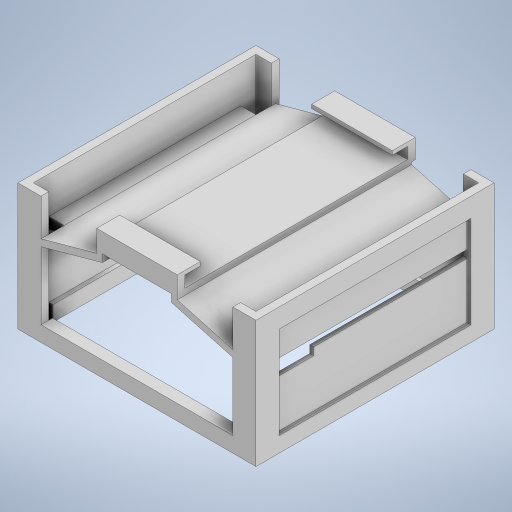
# Autodesk Inventor part: Unterbau V3
Saved by Autodesk Inventor 2023.1 (Build 271208000, 208)
## iProperties
Created: 2023-04-17
Part Number: Unterbau V3
Material: Generisch
Document SubType Name: Modeling
Designer: marco
Density: 1 g/cm^3
Appearance: Vorgabe
Author: marco
Autodesk Inventor part; units mm, degrees
ref_plane "YZ Plane" through (0, 0, 0) normal (1, 0, 0) x (0, 1, 0)
ref_plane "XZ Plane" through (0, 0, 0) normal (0, 1, 0) x (-1, 0, 0)
ref_plane "XY Plane" through (0, 0, 0) normal (0, 0, 1) x (1, 0, 0)
sketch "Skizze1" plane through (0, 0, 0) normal (0, 1, 0) x (-1, 0, 0)
  line L0 (0, 0) -> (62, 0)
  line L1 (62, 0) -> (62, -62)
  line L2 (62, -62) -> (0, -62)
  line L3 (0, -62) -> (0, 0)
  line L4 (2, -2) -> (6, -2)
  line L5 (6, -2) -> (6, -6)
  line L6 (6, -6) -> (2, -6)
  line L7 (2, -6) -> (2, -2)
  line L8 (2, -56) -> (6, -56)
  line L9 (6, -56) -> (6, -60)
  line L10 (6, -60) -> (2, -60)
  line L11 (2, -60) -> (2, -56)
  line L12 (56, -2) -> (60, -2)
  line L13 (60, -2) -> (60, -6)
  line L14 (60, -6) -> (56, -6)
  line L15 (56, -6) -> (56, -2)
  line L16 (56, -56) -> (60, -56)
  line L17 (60, -56) -> (60, -60)
  line L18 (60, -60) -> (56, -60)
  line L19 (56, -60) -> (56, -56)
  line L20 (3, -3) -> (59, -3)
  line L21 (59, -3) -> (59, -59)
  line L22 (59, -59) -> (3, -59)
  line L23 (3, -59) -> (3, -3)
  point P0 (2, -58)
  point P1 (6, -3)
  point P2 (56, -3)
  point P3 (59, -6)
  point P4 (59, -56)
  point P5 (56, -59)
  point P6 (6, -59)
  point P7 (3, -56)
  point P8 (3, -6)
  dimension "d0" = 62
  dimension "d1" = 62
  dimension "d2" = 4
  dimension "d3" = 4
  dimension "d4" = 4
  dimension "d5" = 4
  dimension "d6" = 4
  dimension "d7" = 50
  dimension "d8" = 50
  dimension "d9" = 2
  dimension "d10" = 2
  dimension "d11" = 2
  dimension "d12" = 56
  dimension "d13" = 56
  constraints: 48 end point, 12 parallel, 7 point on line, 6 horizontal, 6 perpendicular, 1 midpoint
  measures "d0" distance of L1.end L2.end
  measures "d1" distance of L0.end L1.end
  measures "d2" distance of L5.end L6.end
  measures "d3" distance of L4.end L5.end
  measures "d4" distance of L9.end L10.end
  measures "d5" distance of L8.end L9.end
  measures "d6" distance of L13.end L14.end
  measures "d7" distance between parallel lines of L15 L5
  measures "d8" distance between parallel lines of L8 L6
  measures "d9" distance between parallel lines of L2 L10
  measures "d10" distance between parallel lines of L1 L17
  measures "d11" distance from line of L3 point (2, -58)
  measures "d12" distance of L21.end L22.end
  measures "d13" distance of L20.end L21.end
extrude "Extrusion1" add sketch "Skizze1" along normal blind 4
sketch "Skizze2" plane through (0, 4, 0) normal (0, 1, 0) x (1, 0, 0)
  line L0 (-2, 2) -> (-6, 2) projected
  line L1 (-3, 6) -> (-2, 6) projected
  line L2 (-6, 2) -> (-2, 2)
  line L3 (-2, 2) -> (-2, 6)
  line L4 (-2, 6) -> (-6, 6)
  line L5 (-6, 6) -> (-6, 2)
  line L6 (-62, 0) -> (0, 0) projected
  line L7 (0, 0) -> (0, 62) projected
  line L8 (-6, 0) -> (0, 0)
  line L9 (0, 0) -> (0, 6)
  line L10 (0, 6) -> (-6, 6)
  line L11 (-6, 6) -> (-6, 0)
  line L12 (0, 62) -> (-62, 62) projected
  line L13 (0, 55.9421) -> (-6, 55.9421)
  line L14 (-6, 55.9421) -> (-6, 62)
  line L15 (-6, 62) -> (0, 62)
  line L16 (0, 62) -> (0, 55.9421)
  line L17 (-6, 59) -> (-6, 60) projected
  line L18 (-6, 60) -> (-2, 60)
  line L19 (-2, 60) -> (-2, 56)
  line L20 (-2, 56) -> (-6, 56)
  line L21 (-6, 56) -> (-6, 60)
  line L22 (-62, 62) -> (-56, 62)
  line L23 (-56, 62) -> (-56, 55.9421)
  line L24 (-56, 55.9421) -> (-62, 55.9421)
  line L25 (-62, 55.9421) -> (-62, 62)
  line L26 (-60, 60) -> (-56, 60) projected
  line L27 (-60, 60) -> (-56, 60)
  line L28 (-56, 60) -> (-56, 55.9421)
  line L29 (-56, 55.9421) -> (-60, 55.9421)
  line L30 (-60, 55.9421) -> (-60, 60)
  line L31 (-62, 62) -> (-62, 0) projected
  line L32 (-62, 6) -> (-56, 6)
  line L33 (-56, 6) -> (-56, 0)
  line L34 (-56, 0) -> (-62, 0)
  line L35 (-62, 0) -> (-62, 6)
  line L36 (-56, 2) -> (-60, 2)
  line L37 (-60, 2) -> (-60, 6)
  line L38 (-60, 6) -> (-56, 6)
  line L39 (-56, 6) -> (-56, 2)
  constraints: 64 end point, 16 parallel, 16 point on line, 8 horizontal, 8 perpendicular
extrude "Extrusion2" add sketch "Skizze2" along normal blind 25 contours L3 L10 L7 L6 L11 L0 | L6 L31 L32 L37 L36 L33 | L13 L14 L20 L19 L18 L12 L7 | L25 L12 L23 L26 L30 L24
sketch "Skizze3" plane through (0, 29, 0) normal (0, 1, 0) x (1, 0, 0)
  line L0 (-62, 0) -> (0, 0) projected
  line L1 (0, 0) -> (-62, 0)
  line L2 (-62, 0) -> (-62, 62)
  line L3 (-62, 62) -> (0, 62)
  line L4 (0, 62) -> (0, 0)
  line L5 (-6, 6) -> (-56, 6)
  line L6 (-56, 6) -> (-56, 56)
  line L7 (-56, 56) -> (-6, 56)
  line L8 (-6, 56) -> (-6, 6)
  line L9 (-60, 2) -> (-60, 6) projected
  line L10 (-56, 6) -> (-60, 6)
  line L11 (-60, 6) -> (-60, 2)
  line L12 (-60, 2) -> (-56, 2)
  line L13 (-56, 2) -> (-56, 6)
  line L14 (-60, 60) -> (-56, 60) projected
  line L15 (-56, 56) -> (-60, 56)
  line L16 (-60, 56) -> (-60, 60)
  line L17 (-60, 60) -> (-56, 60)
  line L18 (-56, 60) -> (-56, 56)
  line L19 (-3, 56) -> (-6, 56) projected
  line L20 (-2, 60) -> (-2, 56) projected
  line L21 (-6, 56) -> (-2, 56)
  line L22 (-2, 56) -> (-2, 60)
  line L23 (-2, 60) -> (-6, 60)
  line L24 (-6, 60) -> (-6, 56)
  line L25 (-2, 2) -> (-6, 2) projected
  line L26 (-6, 6) -> (-2, 6)
  line L27 (-2, 6) -> (-2, 2)
  line L28 (-2, 2) -> (-6, 2)
  line L29 (-6, 2) -> (-6, 6)
  dimension "d18" = 50
  dimension "d19" = 50
  constraints: 48 end point, 12 parallel, 6 horizontal, 6 perpendicular
  measures "d18" distance of L6.end L7.end
  measures "d19" distance of L5.end L6.end
extrude "Extrusion3" add sketch "Skizze3" along normal blind 4
sketch "Skizze4" plane through (0, 29, 0) normal (0, -1, 0) x (1, 0, 0)
  line L0 (-6, -6) -> (-56, -6) projected
  line L1 (-6, -6) -> (-2, -6)
  line L2 (-2, -6) -> (-2, -56)
  line L3 (-2, -56) -> (-6, -56)
  line L4 (-6, -56) -> (-6, -6)
  line L5 (-6, -56) -> (-56, -56)
  line L6 (-56, -56) -> (-56, -60)
  line L7 (-56, -60) -> (-6, -60)
  line L8 (-6, -60) -> (-6, -56)
  line L9 (-56, -6) -> (-56, -2) projected
  line L10 (-56, -6) -> (-6, -6)
  line L11 (-6, -6) -> (-6, -2)
  line L12 (-6, -2) -> (-56, -2)
  line L13 (-56, -2) -> (-56, -6)
  line L14 (-60, -6) -> (-56, -6) projected
  line L15 (-56, -6) -> (-60, -6)
  line L16 (-60, -6) -> (-60, -56)
  line L17 (-60, -56) -> (-56, -56)
  line L18 (-56, -56) -> (-56, -6)
  point P0 (0, 0)
  dimension "d22" = 4
  dimension "d23" = 50
  dimension "d24" = 50
  dimension "d25" = 4
  dimension "d26" = 50
  dimension "d27" = 4
  dimension "d28" = 4
  dimension "d29" = 50
  constraints: 32 end point, 8 parallel, 4 horizontal, 4 perpendicular
  measures "d22" distance of L2.end L3.end
  measures "d23" distance of L1.end L2.end
  measures "d24" distance of L7.end L6.end
  measures "d25" distance of L6.end L5.end
  measures "d26" distance of L12.end L11.end
  measures "d27" distance of L11.end L10.end
  measures "d28" distance of L17.end L16.end
  measures "d29" distance of L16.end L15.end
extrude "Extrusion4" cut sketch "Skizze4" against normal blind 2 contours L1 L2 L3 L4 | L0 L9 L12 L11 | L18 L17 L16 L14 | L8 L7 L6 L5
sketch "Skizze5" plane through (0, 31, 0) normal (0, -1, 0) x (1, 0, 0)
  line L0 (-59, -59) -> (-3, -59)
  line L1 (-3, -59) -> (-3, -3)
  line L2 (-59, -3) -> (-59, -59)
  line L3 (-57.5, -4.5) -> (-57.5, -57.5)
  line L4 (-57.5, -57.5) -> (-4.5, -57.5)
  line L5 (-4.5, -57.5) -> (-4.5, -4.5)
  line L6 (-62, 0) -> (0, 0) projected
  line L7 (0, 0) -> (0, -62) projected
  line L8 (-60, -60) -> (-56, -60) projected
  line L9 (-2, -6) -> (-2, -2) projected
  line L10 (-60, -60) -> (-2, -60)
  line L11 (-2, -60) -> (-2, -2)
  line L12 (-2, -2) -> (-60, -2)
  line L13 (-60, -2) -> (-60, -60)
  dimension "d32" = 56
  dimension "d33" = 56
  dimension "d34" = 53
  dimension "d35" = 53
  dimension "d36" = 1.5
  dimension "d39" = 3
  constraints: 20 end point, 4 parallel, 2 horizontal, 2 perpendicular
  measures "d32" distance of L2.start L1.end
  measures "d33" distance of L1.end L0.end
  measures "d34" distance of L4.end L3.end
  measures "d35" distance of L3.end L3.start
  measures "d36" distance between parallel lines of L5 L1
  measures "d39" distance between parallel lines of L1 L7
extrude "Extrusion5" cut sketch "Skizze5" against normal blind 1
sketch "Skizze6" plane through (0, 32, 0) normal (0, -1, 0) x (1, 0, 0)
  line L0 (-60, -6) -> (-56, -6) projected
  line L1 (-56, -6) -> (-52, -6)
  line L2 (-6, -6) -> (-56, -6) projected
  line L3 (-52, -6) -> (-56, -10)
  line L4 (-56, -6) -> (-56, -56) projected
  line L5 (-56, -10) -> (-56, -6)
  line L6 (-6, -56) -> (-6, -6) projected
  line L7 (-6, -6) -> (-10, -6)
  line L8 (-6, -6) -> (-2, -6) construction
  line L9 (-10, -6) -> (-6, -10)
  line L10 (-6, -10) -> (-6, -6)
  line L11 (-6, -56) -> (-6, -60) projected
  line L12 (-6, -56) -> (-6, -52)
  line L13 (-6, -52) -> (-10, -56)
  line L14 (-56, -56) -> (-6, -56) projected
  line L15 (-56, -56) -> (-52, -56)
  line L16 (-56, -52) -> (-52, -56)
  line L17 (-56, -52) -> (-56, -56)
  point P0 (0, 0)
  dimension "d42" = 4
  dimension "d43" = 45
  dimension "d44" = 4
  dimension "d45" = 180
  constraints: 24 end point, 6 point on line, 4 collinear, 2 perpendicular, 1 horizontal
  measures "d42" distance of L0.end L1.end
  measures "d43" angle of L1 L3
  measures "d44" distance of L2.start L7.end
  measures "d45" angle of L7 L8
extrude "Extrusion6" add sketch "Skizze6" against normal blind 1 contours L1 L3 L4 | L2 L6 L9 | L16 L14 L4 | L6 L14 L13
sketch "Skizze7" plane through (-6, 4, -55.9421) normal (0, 0, 1) x (1, 0, 0)
  line L0 (3, 0) -> (0, 0) projected
  line L1 (0, 0) -> (4, 0)
  line L2 (4, 0) -> (4, 25)
  line L3 (4, 25) -> (0, 25)
  line L4 (0, 25) -> (0, 0)
  point P0 (6, -4)
  constraints: 8 end point, 2 parallel, 1 horizontal, 1 perpendicular
extrude "Extrusion7" cut sketch "Skizze7" against normal blind 1
sketch "Skizze10" plane through (0, 29, 0) normal (0, -1, 0) x (1, 0, 0)
  line L0 (-2, -6) -> (-2, -55.9421) projected
  line L1 (-6, -6) -> (-2, -6) projected
  line L2 (-2, -6) -> (-6, -6)
  line L3 (-6, -2) -> (-6, -6) projected
  line L4 (-6, -6) -> (-6, -2)
  line L5 (-56, -3) -> (-56, -2) projected
  line L6 (-6, -2) -> (-56, -2)
  line L7 (-56, -6) -> (-56, -2) projected
  line L8 (-56, -2) -> (-56, -6)
  line L9 (-60, -6) -> (-56, -6) projected
  line L10 (-56, -6) -> (-60, -6)
  line L11 (-60, -56) -> (-60, -60) projected
  line L12 (-60, -6) -> (-60, -56)
  line L13 (-56, -56) -> (-60, -56) projected
  line L14 (-60, -56) -> (-56, -56)
  line L15 (-56, -60) -> (-56, -56) projected
  line L16 (-56, -56) -> (-56, -60)
  line L17 (-6, -59) -> (-6, -60) projected
  line L18 (-56, -60) -> (-6, -60)
  line L19 (-6, -56) -> (-6, -60) projected
  line L20 (-6, -60) -> (-6, -56)
  line L21 (-3, -56) -> (-2, -56) projected
  line L22 (-6, -56) -> (-2, -56)
  line L23 (-2, -56) -> (-2, -6)
  line L24 (0, -6) -> (0, -55.9421) projected
  line L25 (-2, -6) -> (0, -6)
  line L26 (0, -6) -> (0, -56)
  line L27 (0, -56) -> (-2, -56)
  line L28 (-6, -62) -> (-56, -62) projected
  line L29 (-6, -60) -> (-6, -62)
  line L30 (-6, -62) -> (-56, -62)
  line L31 (-56, -62) -> (-56, -60)
  line L32 (-56, 0) -> (-6, 0) projected
  line L33 (-56, -2) -> (-56, 0)
  line L34 (-56, 0) -> (-6, 0)
  line L35 (-6, -2) -> (-6, 0) projected
  line L36 (-6, 0) -> (-6, -2)
  line L37 (-60, -6) -> (-62, -6)
  line L38 (-62, -62) -> (-62, 0) projected
  line L39 (-62, -56) -> (-62, -6)
  line L40 (-59, -6) -> (-59, -56) projected
  line L41 (-62, -56) -> (-60, -56)
  point P0 (0, 0)
  constraints: 48 end point, 11 perpendicular, 8 collinear, 2 horizontal, 2 point on line, 2 vertical, 1 parallel
extrude "Extrusion8" add sketch "Skizze10" along normal blind 1
sketch "Skizze11" plane through (0, 0, 0) normal (0, -1, 0) x (1, 0, 0)
  line L0 (-60, -60) -> (-56, -60) projected
  line L1 (-2, -6) -> (-2, -2) projected
  line L2 (-60, -60) -> (-2, -60)
  line L3 (-2, -60) -> (-2, -2)
  line L4 (-2, -2) -> (-60, -2)
  line L5 (-60, -2) -> (-60, -60)
  line L6 (-1, -1) -> (-61, -1)
  line L7 (-61, -1) -> (-61, -61)
  line L8 (-61, -61) -> (-1, -61)
  line L9 (-1, -61) -> (-1, -1)
  point P0 (0, 0)
  dimension "d52" = 60
  dimension "d53" = 60
  constraints: 16 end point, 4 parallel, 2 horizontal, 2 perpendicular
  measures "d52" distance of L8.end L7.end
  measures "d53" distance of L7.end L6.end
extrude "Extrusion9" add sketch "Skizze11" against normal blind 28
sketch "Skizze13" plane through (-56, 28, -1) normal (0, 0, 1) x (1, 0, 0)
  line L0 (0, -24) -> (50, -24) projected
  line L1 (0, 0) -> (-4, 0) projected
  line L2 (50, -24) -> (0, -24)
  line L3 (0, -24) -> (0, 0)
  line L4 (0, 0) -> (50, 0)
  line L5 (50, 0) -> (50, -24)
  point P0 (56, -28)
  constraints: 8 end point, 2 parallel, 1 horizontal, 1 perpendicular
extrude "Extrusion10" cut sketch "Skizze13" against normal blind 1
sketch "Skizze16" plane through (-1, 4, -55.9421) normal (1, 0, 0) x (0, 0, -1)
  line L0 (0, 24) -> (0, 0) projected
  line L1 (-49.9421, 0) -> (-49.9421, 24) projected
  line L2 (0, 16.5) -> (-49.9421, 16.5)
  line L3 (-49.9421, 16.5) -> (-49.9421, 14.5)
  line L4 (-49.9421, 14.5) -> (0, 14.5)
  line L5 (0, 14.5) -> (0, 16.5)
  point P0 (-55.9421, -4)
  point P1 (-49.9421, 16.5)
  dimension "d67" = 2
  constraints: 8 end point, 2 parallel, 2 point on line, 1 horizontal, 1 perpendicular
  measures "d67" distance of L3.end L2.end
extrude "Extrusion13" cut sketch "Skizze16" against normal blind 5
sketch "Skizze18" plane through (-62, 0, 0) normal (0, 0, 1) x (1, 0, 0)
  line L0 (2, 28) -> (6, 28) projected
  line L1 (2, 28) -> (22, 28)
  line L2 (2, 28) -> (22, 28) construction
  line L3 (22, 28) -> (22, 26)
  line L4 (56, 28) -> (60, 28) projected
  line L5 (60, 28) -> (40, 28)
  line L6 (6, 28) -> (56, 28) projected
  line L7 (40, 28) -> (40, 26)
  line L8 (61, 20.5) -> (60, 20.5) projected
  line L9 (40, 26) -> (60, 20.5)
  line L10 (60, 20.5) -> (60, 28)
  line L11 (22, 26) -> (2, 20.5)
  line L12 (2, 0) -> (2, 33) projected
  line L13 (2, 28) -> (2, 20.5)
  point P0 (62, 0)
  dimension "d71" = 20
  dimension "d72" = 0
  dimension "d73" = 2
  dimension "d74" = 20
  constraints: 18 end point, 2 horizontal, 2 parallel, 2 perpendicular, 2 point on line, 1 collinear
  measures "d71" distance of L0.start L1.end
  measures "d72" distance between parallel lines of L1 L2
  measures "d73" distance of L1.end L3.end
  measures "d74" distance of L4.end L5.end
extrude "Extrusion14" add sketch "Skizze18" against normal blind 60
sketch "Skizze19" plane through (-62, 0, 0) normal (0, 0, 1) x (1, 0, 0)
  line L0 (56, 23.3797) -> (56, 33)
  line L1 (0, 33) -> (62, 33) projected
  line L2 (56, 33) -> (52, 33) projected
  line L3 (56, 33) -> (41.5, 33)
  line L4 (52, 33) -> (10, 33) projected
  line L5 (56, 33) -> (70.5, 33) construction
  line L6 (41.5, 33) -> (41.5, 27.3672)
  line L7 (56, 28) -> (6, 28) projected
  line L8 (41.5, 27.3672) -> (56, 23.3797)
  line L9 (40, 26) -> (56, 21.6) projected
  line L10 (6, 28) -> (6, 4) projected
  line L11 (6, 23.3797) -> (6, 33)
  line L12 (10, 33) -> (6, 33) projected
  line L13 (6, 33) -> (20.5, 33)
  line L14 (20.5, 33) -> (20.5, 27.3672)
  line L15 (20.5, 27.3672) -> (6, 23.3797)
  point P0 (62, 0)
  dimension "d77" = 14.5
  dimension "d78" = 180
  dimension "d79" = 14.5
  constraints: 18 end point, 4 point on line, 3 perpendicular, 2 collinear, 1 horizontal, 1 parallel, 1 vertical
  measures "d77" distance of L0.end L3.end
  measures "d78" angle of L3 L5
  measures "d79" distance of L11.end L13.end
extrude "Extrusion15" cut sketch "Skizze19" against normal blind 71.1125 contours L8 L6 L7 L0 | L7 L6 L1 L0 | L14 L15 L10 L7 | L7 L11 L1 L14
sketch "Skizze20" plane through (-1, 4, -6) normal (1, 0, 0) x (0, 0, -1)
  line L0 (0, 16.5) -> (49.9421, 16.5) projected
  line L1 (0, 16.5) -> (10, 16.5)
  line L2 (10, 16.5) -> (10, 12.5)
  line L3 (10, 12.5) -> (0, 12.5)
  line L4 (0, 12.5) -> (0, 16.5)
  point P0 (-6, -4)
  dimension "d82" = 10
  dimension "d83" = 4
  constraints: 8 end point, 2 parallel, 1 horizontal, 1 perpendicular
  measures "d82" distance of L2.end L3.end
  measures "d83" distance of L1.end L2.end
extrude "Extrusion16" cut sketch "Skizze20" against normal blind 2
sketch "Skizze21" plane through (0, 33, 0) normal (0, 1, 0) x (1, 0, 0)
  line L0 (-1, 6) -> (-2, 6) projected
  line L1 (-6, 0) -> (-6, 2) projected
  line L2 (-2, 6) -> (-6, 6)
  line L3 (-6, 6) -> (-6, 2)
  line L4 (-6, 2) -> (-2, 2)
  line L5 (-2, 2) -> (-2, 6)
  line L6 (-56, 2) -> (-60, 2)
  line L7 (-60, 2) -> (-60, 6)
  line L8 (-60, 6) -> (-56, 6)
  line L9 (-56, 6) -> (-56, 2)
  line L10 (-60, 56) -> (-60, 60) projected
  line L11 (-60, 60) -> (-56, 60) projected
  line L12 (-60, 56) -> (-56, 56)
  line L13 (-56, 56) -> (-56, 60)
  line L14 (-56, 60) -> (-60, 60)
  line L15 (-60, 60) -> (-60, 56)
  line L16 (-6, 60) -> (-2, 60) projected
  line L17 (-6, 56) -> (-2, 56) projected
  line L18 (-2, 60) -> (-6, 60)
  line L19 (-6, 60) -> (-6, 56)
  line L20 (-6, 56) -> (-2, 56)
  line L21 (-2, 56) -> (-2, 60)
  point P0 (0, 0)
  constraints: 32 end point, 8 parallel, 4 horizontal, 4 perpendicular
extrude "Extrusion17" cut sketch "Skizze21" against normal blind 20
sketch "Skizze22" plane through (-60, 29, -6) normal (0, 0, 1) x (1, 0, 0)
  line L0 (54, 0) -> (54, -5.6203) projected
  line L1 (58, 3) -> (58, 4) projected
  line L2 (54, -5.6203) -> (58, -5.6203)
  line L3 (58, -5.6203) -> (58, 4)
  line L4 (58, 4) -> (54, 4)
  line L5 (54, 4) -> (54, -5.6203)
  line L6 (4, 0) -> (4, -5.6203) projected
  line L7 (0, -29) -> (0, 4) projected
  line L8 (4, -5.6203) -> (0, -5.6203)
  line L9 (0, -5.6203) -> (0, 4)
  line L10 (0, 4) -> (4, 4)
  line L11 (4, 4) -> (4, -5.6203)
  point P0 (60, -29)
  constraints: 16 end point, 4 parallel, 2 horizontal, 2 perpendicular
extrude "Extrusion18" cut sketch "Skizze22" against normal blind 51.4375
